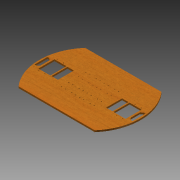
# Autodesk Inventor part: ChassisRound
Saved by Autodesk Inventor 2014 SP1 (Build 180222100, 222)
## iProperties
Created: 2015-03-16
Part Number: ChassisRound
Material: Wood (Oak)
Document SubType Name: Modeling
Designer: david
Density: 0.76 g/cm^3
Appearance: Yellow Pine - Solid Stained Light Low Gloss
Mass: 358.304 g
Surface Area: 1717.54 cm^2
Volume: 471.453 cm^3
Author: david
Autodesk Inventor part; units mm, degrees
ref_plane "YZ Plane" through (0, 0, 0) normal (1, 0, 0) x (0, 1, 0)
ref_plane "XZ Plane" through (0, 0, 0) normal (0, 1, 0) x (-1, 0, 0)
ref_plane "XY Plane" through (0, 0, 0) normal (0, 0, 1) x (1, 0, 0)
sketch "BodySketch" plane through (0, 0, 0) normal (0, 1, 0) x (-1, 0, 0)
  line L0 (0, 125) -> (143.0909, 125)
  line L1 (143.0909, -125) -> (0, -125)
  line L2 (0, 0) -> (0, 145.614) construction
  line L3 (0, 125) -> (-143.0909, 125)
  line L4 (-143.0909, -125) -> (0, -125)
  line L5 (0, 0) -> (316.974, 0) construction
  arc A0 (143.0909, -125) -> (143.0909, 125) centre (0, 0) ccw
  arc A1 (-143.0909, 125) -> (-143.0909, -125) centre (0, 0) ccw
  dimension "Chassis_Body_Length" = 250
  dimension "d76" = 190
  constraints: 12 end point, 4 point on circle, 3 parallel, 2 centre point, 2 point on line, 2 symmetric about line, 1 coincident, 1 horizontal, 1 perpendicular, 1 other
  measures "Chassis_Body_Length" distance between parallel lines of L1 L0
  measures "d76" radius of A0
extrude "Body" add sketch "BodySketch" along normal blind 6
sketch "EncoderWheelHoleSketch" plane through (0, 6, 0) normal (0, 1, 0) x (1, 0, 0)
  line L0 (-169.5, 18) -> (-169.5, -18)
  line L1 (-184, -24.5) -> (-184, 24.5)
  line L2 (-143.0909, -125) -> (143.0909, -125) projected
  arc A0 (-143.0909, 125) -> (-143.0909, -125) centre (0, 0) ccw projected
  line L3 (-184, 24.5) -> (-178, 24.5)
  line L4 (-178, 24.5) -> (-169.5, 18)
  line L5 (-169.5, -18) -> (-178, -24.5)
  line L6 (-178, -24.5) -> (-184, -24.5)
  line L7 (0, 0) -> (-101.7765, 0) construction
  line L8 (0, 0) -> (0, 68.8757) construction
  line L9 (169.5, 18) -> (169.5, -18)
  line L10 (184, -24.5) -> (184, 24.5)
  line L11 (184, 24.5) -> (178, 24.5)
  line L12 (178, 24.5) -> (169.5, 18)
  line L13 (169.5, -18) -> (178, -24.5)
  line L14 (178, -24.5) -> (184, -24.5)
  point P0 (-190, 0)
  dimension "d80" = 6
  dimension "d81" = 14.5
  dimension "d82" = 49
  dimension "d83" = 36
  dimension "d84" = 6
  constraints: 28 end point, 7 symmetric about line, 5 parallel, 1 perpendicular, 1 point on circle, 1 point on line, 1 other
  measures "d80" distance of L1.end L3.end
  measures "d81" distance between parallel lines of L0 L1
  measures "d82" distance between parallel lines of L6 L3
  measures "d83" distance of L0.start L0.end
  measures "d84" distance from line of point (-190, 0) L1
extrude "EncoderWheelHole" cut sketch "EncoderWheelHoleSketch" against normal up to next
sketch "EncoderBodyHoleSketch" plane through (0, 6, 0) normal (0, 1, 0) x (1, 0, 0)
  line L0 (0, 0) -> (0, 145.3586) construction
  line L1 (-163.5, 30.25) -> (-118.5, 30.25)
  line L2 (-118.5, 30.25) -> (-118.5, -30.25)
  line L3 (-118.5, -30.25) -> (-163.5, -30.25)
  line L4 (-163.5, -30.25) -> (-163.5, 30.25)
  line L5 (0, 0) -> (187.4589, 0) construction
  line L6 (163.5, 30.25) -> (118.5, 30.25)
  line L7 (118.5, 30.25) -> (118.5, -30.25)
  line L8 (118.5, -30.25) -> (163.5, -30.25)
  line L9 (163.5, -30.25) -> (163.5, 30.25)
  line L10 (-141, -22.1441) -> (-141, 50.5352) construction
  line L11 (-169.5, 18) -> (-169.5, -18) projected
  line L12 (-184, -24.5) -> (-184, 24.5) projected
  dimension "d9" = 45
  dimension "d10" = 60.5
  dimension "d85" = 43
  constraints: 22 end point, 4 symmetric about line, 3 parallel, 2 perpendicular, 1 horizontal, 2 other
  measures "d9" distance between parallel lines of L2 L4
  measures "d10" distance between parallel lines of L3 L1
  measures "d85" distance between parallel lines of L12 L10
extrude "EncoderBodyHole" cut sketch "EncoderBodyHoleSketch" against normal up to next
sketch "EncoderSupportFasteningSketch" plane through (0, 6, 0) normal (0, 1, 0) x (1, 0, 0)
  line L0 (-129.5, 39.75) -> (-162.5, 39.75) construction
  line L1 (-162.5, 39.75) -> (-162.5, -39.75) construction
  line L2 (-129.5, -39.75) -> (-129.5, 39.75) construction
  circle A0 centre (-157.5, 34.75) radius 1.5
  line L3 (-146, 46.4919) -> (-146, -51.9033) construction
  circle A1 centre (-134.5, 34.75) radius 1.5
  line L4 (0, 0) -> (78.2402, 0) construction
  circle A2 centre (-157.5, -34.75) radius 1.5
  circle A3 centre (-134.5, -34.75) radius 1.5
  line L5 (-162.5, -39.75) -> (-129.5, -39.75) construction
  line L6 (0, 0) -> (0, 64.4845) construction
  circle A4 centre (157.5, 34.75) radius 1.5
  circle A5 centre (134.5, 34.75) radius 1.5
  circle A6 centre (157.5, -34.75) radius 1.5
  circle A7 centre (134.5, -34.75) radius 1.5
  line L7 (-184, -24.5) -> (-184, 24.5) projected
  dimension "d17" = 33
  dimension "d19" = 3
  dimension "d20" = 5
  dimension "d21" = 5
  dimension "d22" = 16.5
  dimension "d69" = 79.5
  dimension "d86" = 21.5
  constraints: 14 end point, 8 centre point, 7 symmetric about line, 2 parallel, 2 perpendicular, 1 horizontal, 8 other
  measures "d17" distance between parallel lines of L1 L2
  measures "d19" diameter of A0
  measures "d20" distance from line of L0 A0.centre
  measures "d21" distance from line of L1 A0.centre
  measures "d22" distance between parallel lines of L1 L3
  measures "d69" distance between parallel lines of L5 L0
  measures "d86" distance between parallel lines of L7 L1
extrude "EncoderSupportFastening" cut sketch "EncoderSupportFasteningSketch" against normal up to next
sketch "MotorBlockFasteningSketch" plane through (0, 6, 0) normal (0, 1, 0) x (1, 0, 0)
  line L0 (10.676, -18) -> (24.3135, -18) construction
  circle A0 centre (7.5, -18) radius 1.5
  circle A1 centre (22.5, -18) radius 1.5
  line L1 (0, 0) -> (0, -28.6489) construction
  circle A2 centre (46.5, -18) radius 1.5
  circle A3 centre (61.5, -18) radius 1.5
  circle A4 centre (7.5, -46) radius 1.5
  circle A5 centre (22.5, -46) radius 1.5
  circle A6 centre (46.5, -46) radius 1.5
  circle A7 centre (61.5, -46) radius 1.5
  circle A8 centre (-7.5, -18) radius 1.5
  circle A9 centre (-22.5, -18) radius 1.5
  circle A10 centre (-46.5, -18) radius 1.5
  circle A11 centre (-61.5, -18) radius 1.5
  circle A12 centre (-7.5, -46) radius 1.5
  circle A13 centre (-22.5, -46) radius 1.5
  circle A14 centre (-46.5, -46) radius 1.5
  circle A15 centre (-61.5, -46) radius 1.5
  line L2 (0, 0) -> (72.0385, 0) construction
  circle A16 centre (7.5, 18) radius 1.5
  circle A17 centre (22.5, 18) radius 1.5
  line L3 (0, 0) -> (0, 28.6489) construction
  circle A18 centre (46.5, 18) radius 1.5
  circle A19 centre (61.5, 18) radius 1.5
  circle A20 centre (7.5, 46) radius 1.5
  circle A21 centre (22.5, 46) radius 1.5
  circle A22 centre (46.5, 46) radius 1.5
  circle A23 centre (61.5, 46) radius 1.5
  circle A24 centre (-7.5, 18) radius 1.5
  circle A25 centre (-22.5, 18) radius 1.5
  circle A26 centre (-46.5, 18) radius 1.5
  circle A27 centre (-46.5, 46) radius 1.5
  circle A28 centre (-61.5, 18) radius 1.5
  circle A29 centre (-61.5, 46) radius 1.5
  circle A30 centre (-7.5, 46) radius 1.5
  circle A31 centre (-22.5, 46) radius 1.5
  dimension "d25" = 3
  dimension "d28" = 15
  dimension "d35" = 39
  dimension "d38" = 28
  dimension "d41" = 15
  dimension "d46" = 18
  constraints: 32 centre point, 25 symmetric about line, 8 end point, 3 horizontal, 1 perpendicular, 1 point on line, 1 vertical, 38 other
  measures "d25" diameter of A0
  measures "d28" distance of A0.centre A1.centre
  measures "d35" distance of A0.centre A2.centre
  measures "d38" distance of A0.centre A4.centre
  measures "d41" distance of A0.centre A8.centre
  measures "d46" distance between parallel lines of L2 L0
extrude "MotorBlockFastening" cut sketch "MotorBlockFasteningSketch" against normal up to next
sketch "MotorWheelHoleSketch" plane through (0, 6, 0) normal (0, 1, 0) x (1, 0, 0)
  line L0 (-114.5, 30) -> (-90.5, 30)
  line L1 (-90.5, 30) -> (-90.5, -30)
  line L2 (-90.5, -30) -> (-114.5, -30)
  line L3 (-114.5, -30) -> (-114.5, 30)
  line L4 (0, 0) -> (64.8732, 0) construction
  line L5 (0, 0) -> (0, 63.2492) construction
  line L6 (-118.5, 30.25) -> (-118.5, -30.25) construction
  line L7 (114.5, 30) -> (90.5, 30)
  line L8 (90.5, 30) -> (90.5, -30)
  line L9 (90.5, -30) -> (114.5, -30)
  line L10 (114.5, -30) -> (114.5, 30)
  dimension "Chassis_MotorWheelHole_Diameter" = 60
  dimension "Chassis_MotorWheelHole_Width" = 24
  dimension "Chassis_MotorWheelHole_DistanceToEncoder" = 4
  constraints: 20 end point, 4 symmetric about line, 3 perpendicular, 2 parallel, 1 horizontal, 1 other
  measures "Chassis_MotorWheelHole_Diameter" distance between parallel lines of L2 L0
  measures "Chassis_MotorWheelHole_Width" distance between parallel lines of L1 L3
  measures "Chassis_MotorWheelHole_DistanceToEncoder" distance between parallel lines of L6 L3
extrude "MotorWheelHole" cut sketch "MotorWheelHoleSketch" against normal up to next
equation "\"d9\" = EncoderSupportInside_Front_Thickness + Encoder_Body_Length + 2 * Chassis_MecanicalSpace"
equation "\"d10\" = EncoderSupportInside_Width + 2 * Chassis_MecanicalSpace"
equation "\"d17\" = EncoderSupportOutside_Length"
equation "\"d19\" = EncoderSupport_FixingHole_Diameter"
equation "\"d20\" = EncoderSupport_FixingnHole_Margin"
equation "\"d21\" = EncoderSupport_FixingnHole_Margin"
equation "\"d22\" = 0.5 * EncoderSupportOutside_Length"
equation "\"d28\" = Bracket_Holes_Distance"
equation "\"d35\" = Bracket_Holes_Distance + Bracket_Holes_UnfoldedDistance"
equation "\"d38\" = Bracket_Holes_LateralDistance"
equation "\"d41\" = Bracket_Holes_Distance"
equation "\"d46\" = Motor_FasteningHole_DistanceToCenter"
equation "\"Chassis_MecanicalSpace\" = 1"
equation "\"EncoderSupportInside_Front_Thickness\" = 3"
equation "\"Encoder_Body_Length\" = 40"
equation "\"EncoderSupportInside_Width\" = 58.5"
equation "\"EncoderSupportOutside_Length\" = 33"
equation "\"EncoderSupport_FixingHole_Diameter\" = 3"
equation "\"EncoderSupport_FixingnHole_Margin\" = 5"
equation "\"Bracket_Holes_Distance\" = 15"
equation "\"Bracket_Holes_UnfoldedDistance\" = 24"
equation "\"Bracket_Holes_LateralDistance\" = 28"
equation "\"Motor_FasteningHole_DistanceToCenter\" = 18"
body "Solid1"
